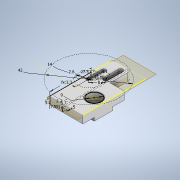
# Autodesk Inventor part: Dreiwegehahn_Montage45
Saved by Autodesk Inventor 2022 (Build 260153000, 153)
## iProperties
Created: 2024-04-03
Part Number: Dreiwegehahn_Montage45
Material: Generic
Document SubType Name: Modeling
Designer: Gotham City
Density: 1 g/cm^3
Appearance: Default
Author: Gotham City
Autodesk Inventor part; units mm, degrees
ref_plane "YZ Plane" through (0, 0, 0) normal (1, 0, 0) x (0, 1, 0)
ref_plane "XZ Plane" through (0, 0, 0) normal (0, 1, 0) x (-1, 0, 0)
ref_plane "XY Plane" through (0, 0, 0) normal (0, 0, 1) x (1, 0, 0)
sketch "Sketch1" plane through (0, 0, 0) normal (1, 0, 0) x (0, 1, 0)
  line L0 (0, 13.75) -> (-5.2, 13.75)
  line L1 (-5.2, 13.75) -> (-5.2, 6.2)
  line L2 (-5.2, 6.2) -> (-7.4, 6.2)
  line L3 (-7.4, 6.2) -> (-7.4, 2.5)
  line L4 (-7.4, 2.5) -> (-13.4, 2.5) construction
  line L5 (-13.4, 2.5) -> (-13.4, -1.6142) construction
  line L6 (-16.08, 0) -> (2.68, 0) construction
  line L7 (0, -13.75) -> (-5.2, -13.75)
  line L8 (-5.2, -13.75) -> (-5.2, -6.2)
  line L9 (-5.2, -6.2) -> (-7.4, -6.2)
  line L10 (-7.4, -6.2) -> (-7.4, -2.5)
  line L11 (-7.4, -2.5) -> (-13.4, -2.5) construction
  line L12 (-13.4, -2.5) -> (-13.4, -1.6142) construction
  line L13 (0, 13.75) -> (0, -13.75)
  line L14 (-7.4, 2.5) -> (-7.4, -2.5)
  point P0 (0, 0)
  dimension "d1" = 5
  dimension "d2" = 3.7
  dimension "d3" = 6
  dimension "d4" = 2.2
  dimension "d5" = 5.2
  dimension "d52" = 27.5
  dimension "d53" = 7.55
  constraints: 28 end point, 6 perpendicular, 6 vertical alignment, 1 horizontal, 1 midpoint, 1 parallel, 1 other
  measures "d1" distance of L11.end L4.end
  measures "d2" distance of L2.end L3.end
  measures "d3" distance of L3.end L4.end
  measures "d4" distance of L1.end L2.end
  measures "d5" distance of L0.start L0.end
  measures "d52" distance between parallel lines of L7 L0
  measures "d53" distance of L0.end L1.end
extrude "Extrusion1" add sketch "Sketch1" along normal blind 22
sketch "Sketch2" plane through (0, -5.2, -13.75) normal (0, 0, -1) x (-1, 0, 0)
  line L0 (0, 0) -> (0, 5.2) projected
  line L1 (0, 5.2) -> (-22, 5.2) projected
  line L2 (-22, 0) -> (-22, 5.2) projected
  line L3 (0, 0) -> (-22, 0) projected
  point P0 (0, 5.2)
extrude "Extrusion2" add sketch "Sketch2" along normal blind 14
sketch "Sketch3" plane through (0, 0, 13.75) normal (0, 1, 0) x (1, 0, 0)
  circle A0 centre (3.3, 22.5) radius 1.3 construction
  circle A1 centre (8.9569, 28.1569) radius 1.55 construction
  line L0 (3.3, 22.5) -> (8.9569, 28.1569) construction
  line L1 (8.9569, 28.1569) -> (2.1344, 28.1569) construction
  line L2 (0, 0) -> (22, 0) construction
  line L3 (22, 41.5) -> (0, 41.5) construction
  line L4 (3.3, 22.5) -> (3.3, 32.5) construction
  line L5 (8.9569, 28.1569) -> (8.9569, 38.1569) construction
  line L6 (0, 0) -> (0, 41.5) projected
  point P0 (0, 13.75)
  point P1 (6.1284, 25.3284)
  point P2 (3.3, 27.5)
  point P3 (0, 19.95)
  point P4 (0, 27.5)
  point P5 (0, 27.5)
  point P6 (0, 27.5)
  dimension "d10" = 2.6
  dimension "d11" = 3.1
  dimension "d12" = 45
  dimension "d17" = 5
  dimension "d43" = 3.3
  dimension "d44" = 8
  dimension "d46" = 0
  constraints: 8 end point, 2 centre point, 2 midpoint, 2 vertical, 1 horizontal, 1 parallel
  measures "d10" diameter of A0
  measures "d11" diameter of A1
  measures "d12" angle of L1 L0
  measures "d17" distance of point (3.3, 27.5) L0.start
  measures "d43" distance from line of L6 L0.start
  measures "d44" distance of L0.start L0.end
  measures "d46" vertical distance of point (0, 27.5) point (3.3, 27.5)
sketch "Sketch4" plane through (0, 0, 13.75) normal (0, 1, 0) x (1, 0, 0)
  line L0 (8.9569, 28.1569) -> (8.9569, 38.1569) construction
  line L1 (3.3, 22.5) -> (3.3, 32.5) construction
  line L2 (8.9569, 28.1569) -> (8.9569, 38.1569) construction
  line L3 (10.5069, 28.1569) -> (10.5069, 38.1569)
  line L4 (7.4069, 38.1569) -> (7.4069, 28.1569)
  arc A0 (7.4069, 28.1569) -> (10.5069, 28.1569) centre (8.9569, 28.1569) ccw
  arc A1 (10.5069, 38.1569) -> (7.4069, 38.1569) centre (8.9569, 38.1569) ccw
  circle A2 centre (8.9569, 28.1569) radius 1.55 construction
  circle A3 centre (3.3, 22.5) radius 1.3 construction
  line L5 (3.3, 22.5) -> (3.3, 32.5) construction
  line L6 (4.6, 22.5) -> (4.6, 32.5)
  line L7 (2, 32.5) -> (2, 22.5)
  arc A4 (2, 22.5) -> (4.6, 22.5) centre (3.3, 22.5) ccw
  arc A5 (4.6, 32.5) -> (2, 32.5) centre (3.3, 32.5) ccw
  point P0 (0, 13.75)
  point P1 (8.9569, 33.1569)
  point P2 (3.3, 27.5)
  constraints: 16 end point, 10 tangent, 8 point on circle, 4 centre point, 4 equal length, 2 midpoint
extrude "Extrusion3" cut sketch "Sketch4" against normal blind 3
sketch "Sketch5" plane through (0, 0, 13.75) normal (0, 1, 0) x (1, 0, 0)
  point P0 (0, 13.75)
ref_plane "Work Plane1" through (0, -2, 13.75) normal (0, 1, 0) x (1, 0, 0)
sketch "Sketch6" plane through (0, -2, 13.75) normal (0, 1, 0) x (1, 0, 0)
  line L0 (0.75, 23.9722) -> (3.3, 25.4445) construction
  line L1 (3.3, 25.4445) -> (5.85, 23.9722) construction
  line L2 (5.85, 23.9722) -> (5.85, 21.0278) construction
  line L3 (5.85, 21.0278) -> (3.3, 19.5555)
  line L4 (0.75, 21.0278) -> (0.75, 23.9722) construction
  line L5 (2, 22.5) -> (2, 32.5) construction
  line L6 (2, 27.5) -> (4.6, 27.5) construction
  line L7 (4.6, 32.5) -> (4.6, 22.5) construction
  line L8 (5.85, 33.9722) -> (3.3, 35.4445)
  line L9 (5.85, 21.0278) -> (5.85, 33.9722)
  line L10 (3.3, 19.5555) -> (0, 19.5555)
  line L11 (0, 7.55) -> (0, 19.95) projected
  line L12 (3.3, 35.4445) -> (0, 35.4445)
  line L13 (0, 0) -> (0, 41.5) projected
  line L14 (0, 19.5555) -> (0, 35.4445)
  point P0 (0, 13.75)
  point P1 (3.3, 22.5)
  point P2 (3.3, 22.5)
  point P3 (3.3, 27.5)
  point P4 (0, 11.25)
  dimension "d21" = 5.1
  constraints: 22 end point, 2 midpoint, 2 point on line, 2 symmetric about line, 2 vertical, 1 coincident, 1 horizontal, 1 parallel, 1 perpendicular, 11 other
  measures "d21" distance between parallel lines of L4 L2
extrude "Extrusion4" cut sketch "Sketch6" against normal through all
sketch "Sketch7" plane through (0, 0, 13.75) normal (0, 1, 0) x (1, 0, 0)
  line L0 (32.7, 13.75) -> (-26.1, 13.75) construction
  circle A0 centre (15.8, 13.75) radius 4.5
  line L1 (22, 0) -> (22, 41.5) projected
  circle A1 centre (3.3, 22.5) radius 7 construction
  line L2 (0, 0) -> (22, 0) construction
  line L3 (10.3, 0) -> (10.3, 41.5) construction
  line L4 (22, 41.5) -> (0, 41.5) construction
  line L5 (11.3, 0) -> (11.3, 41.5) construction
  point P0 (0, 13.75)
  dimension "d24" = 9
  dimension "d39" = 14
  dimension "d41" = 1
  constraints: 4 end point, 4 point on line, 2 centre point, 2 tangent, 1 coincident, 1 perpendicular, 1 vertical, 2 other
  measures "d24" diameter of A0
  measures "d39" diameter of A1
  measures "d41" distance between parallel lines of L3 L5
hole "Hole1" at (15.8, 0, 0) direction (0, -1, 0) diameter 5.5 end through all counterbore diameter 10 counterbore depth 5 clearance for "Socket Head Cap Screw ISO 4762" size "M5" standard "ISO"
sketch "Sketch9" plane through (0, 0, 13.75) normal (0, 1, 0) x (1, 0, 0)
  line L0 (22, 19.95) -> (22, 41.5) projected
  line L1 (22, 27.5) -> (12.5069, 27.5)
  line L2 (12.5069, 27.5) -> (12.5069, 41.5)
  line L3 (12.5069, 41.5) -> (22, 41.5)
  line L4 (22, 41.5) -> (22, 27.5)
  line L5 (10.5069, 38.1569) -> (10.5069, 28.1569) projected
  line L6 (0, 41.5) -> (22, 41.5) projected
  point P0 (0, 13.75)
  point P1 (10.5069, 37.5)
  point P2 (0, 27.5)
  point P3 (0, 27.5)
  point P4 (0, 27.5)
  dimension "d45" = 2
  constraints: 8 end point, 2 parallel, 2 point on line, 1 horizontal, 1 perpendicular, 2 other
  measures "d45" distance between parallel lines of L5 L2
extrude "Extrusion6" cut sketch "Sketch9" against normal through all
fillet "Fillet1" radius 2 1 edges at (12.5069, -2.6, -27.75)
fillet "Fillet2" radius 2 1 edges at (0, -2.6, -27.75)
sketch "Sketch10" plane through (0, 0, 13.75) normal (0, 1, 0) x (1, 0, 0)
  circle A0 centre (3.3, 22.5) radius 21 construction
  point P0 (0, 13.75)
  dimension "d51" = 42
  constraints: 1 centre point, 1 coincident
  measures "d51" diameter of A0
body "Solid1"
